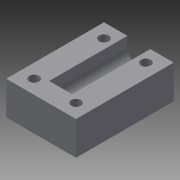
# Autodesk Inventor part: roll_mount2
Saved by Autodesk Inventor 2013 (Build 170138000, 138)
## iProperties
Created: 2014-02-21
Part Number: roll_mount2
Material: Ogólny
Document SubType Name: Modeling
Designer: Piotr
Density: 1 g/cm^3
Author: Piotr
Autodesk Inventor part; units mm, degrees
ref_plane "YZ Plane" through (0, 0, 0) normal (1, 0, 0) x (0, 1, 0)
ref_plane "XZ Plane" through (0, 0, 0) normal (0, 1, 0) x (-1, 0, 0)
ref_plane "XY Plane" through (0, 0, 0) normal (0, 0, 1) x (1, 0, 0)
sketch "Szkic1" plane through (0, 0, 0) normal (0, 0, 1) x (1, 0, 0)
  line L0 (-12.5, -17.5) -> (12.5, -17.5)
  line L1 (12.5, -17.5) -> (12.5, 17.5)
  line L2 (12.5, 17.5) -> (-12.5, 17.5)
  line L3 (-12.5, 17.5) -> (-12.5, -17.5)
  line L4 (-12.5, -17.5) -> (12.5, 17.5) construction
  line L5 (12.5, -17.5) -> (-12.5, 17.5) construction
  line L6 (7.5, -12.5) -> (-7.5, -12.5) construction
  line L7 (-7.5, -12.5) -> (-7.5, 12.5) construction
  line L8 (-7.5, 12.5) -> (7.5, 12.5) construction
  line L9 (7.5, 12.5) -> (7.5, -12.5) construction
  line L10 (7.5, -12.5) -> (-7.5, 12.5) construction
  line L11 (-7.5, -12.5) -> (7.5, 12.5) construction
  point P0 (0, 0)
  dimension "d0" = 25
  dimension "d1" = 35
  dimension "d2" = 15
  dimension "d3" = 25
  constraints: 24 end point, 4 coincident, 4 midpoint, 4 parallel, 2 horizontal, 2 perpendicular
  measures "d0" distance of L2.end L1.end
  measures "d1" distance of L1.end L0.end
  measures "d2" distance of L7.end L8.end
  measures "d3" distance of L6.end L7.end
extrude "Wyciągnięcie proste1" add sketch "Szkic1" along normal blind 12
hole "Otwór1" at (-7.5, 12.5, 0) at (7.5, 12.5, 0) at (7.5, -12.5, 0) at (-7.5, -12.5, 0) direction (0, 0, 1) diameter 3.5 end through all
sketch "Szkic2" plane through (-12.5, 17.5, 0) normal (0, 1, 0) x (1, 0, 0)
  line L0 (25, -12) -> (0, -12) projected
  line L1 (12.5, 0) -> (12.5, -12) construction
  line L2 (8.4, -12) -> (8.4, -8.5)
  arc A0 (16.6, -8.5) -> (8.4, -8.5) centre (12.5, -8.5) ccw
  line L3 (16.6, -8.5) -> (16.6, -12)
  dimension "d13" = 4.1
  dimension "d15" = 3.5
  constraints: 6 end point, 3 point on line, 2 perpendicular, 2 point on circle, 2 tangent, 1 centre point, 1 midpoint
  measures "d13" radius of A0
  measures "d15" distance of L3.start L3.end
extrude "Wyciągnięcie proste2" cut sketch "Szkic2" against normal blind 28
